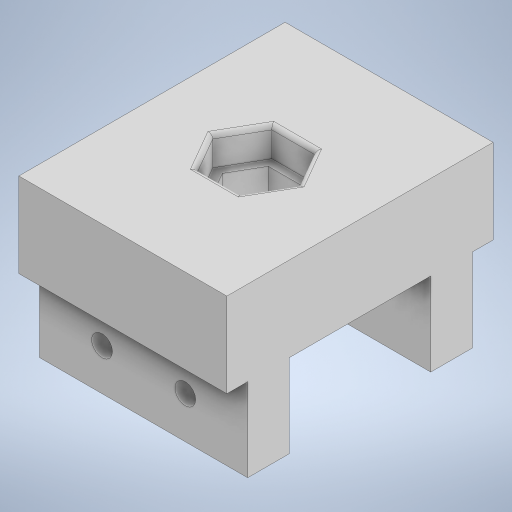
# Autodesk Inventor part: Tensile_test_bottom_adapter2
Saved by Autodesk Inventor 2024 (Build 280153000, 153)
## iProperties
Created: 2023-10-26
Part Number: Tensile_test_bottom_adapter2
Material: 일반
Document SubType Name: Modeling
Designer: jsw
Density: 1 g/cm^3
Appearance: 기본값
Author: jsw
Autodesk Inventor part; units mm, degrees
ref_plane "YZ Plane" through (0, 0, 0) normal (1, 0, 0) x (0, 1, 0)
ref_plane "XZ Plane" through (0, 0, 0) normal (0, 1, 0) x (-1, 0, 0)
ref_plane "XY Plane" through (0, 0, 0) normal (0, 0, 1) x (1, 0, 0)
sketch "스케치1" plane through (0, 0, 0) normal (0, 1, 0) x (-1, 0, 0)
  line L0 (-12.5, 16) -> (12.5, 16)
  line L1 (12.5, 16) -> (12.5, -16)
  line L2 (12.5, -16) -> (-12.5, -16)
  line L3 (-12.5, -16) -> (-12.5, 16)
  line L4 (-12.5, 16) -> (12.5, -16) construction
  line L5 (12.5, 16) -> (-12.5, -16) construction
  point P0 (0, 0)
  dimension "d0" = 25
  dimension "d1" = 32
  constraints: 12 end point, 2 midpoint, 2 parallel, 1 horizontal, 1 perpendicular
  measures "d0" distance of L1.end L2.end
  measures "d1" distance of L0.end L1.end
extrude "돌출1" add sketch "스케치1" along normal blind 10.16
sketch "스케치4" plane through (0, 0, 0) normal (0, -1, 0) x (1, 0, 0)
  line L0 (-12.5, -16) -> (-12.5, 16) projected
  line L1 (12.5, 16) -> (12.5, -16) projected
  line L2 (-12.5, 13.5) -> (12.5, 13.5)
  line L3 (12.5, 13.5) -> (12.5, 8.5)
  line L4 (12.5, 8.5) -> (-12.5, 8.5)
  line L5 (-12.5, 8.5) -> (-12.5, 13.5)
  line L6 (-12.5, 0) -> (12.5, 0)
  line L7 (-12.5, 16) -> (-12.5, -16)
  line L8 (12.5, -10.8) -> (12.5, 10.8)
  line L9 (-12.5, -13.5) -> (12.5, -13.5)
  line L10 (12.5, -13.5) -> (12.5, -8.5)
  line L11 (12.5, -8.5) -> (-12.5, -8.5)
  line L12 (-12.5, -8.5) -> (-12.5, -13.5)
  point P0 (0, 0)
  point P1 (12.5, -8.5)
  point P2 (-12.5, -13.5)
  point P3 (12.5, -13.5)
  point P4 (12.5, 13.5)
  dimension "d13" = 8.5
  dimension "d14" = 5
  constraints: 22 end point, 8 symmetric about line, 4 point on line, 2 midpoint, 2 parallel, 1 horizontal, 1 perpendicular
  measures "d13" distance from line of point (0, 0) L4
  measures "d14" distance of L2.end L3.end
extrude "돌출4" add sketch "스케치4" along normal blind 10 contours L0 L11 L1 L9 | L0 L2 L1 L4
sketch "스케치5" plane through (12.5, 0, -13.5) normal (0, 0, -1) x (-1, 0, 0)
  circle A0 centre (17.5, -5) radius 1.25
  line L0 (25, -10) -> (0, -10) projected
  line L1 (25, 0) -> (25, -10) projected
  line L2 (12.5, -10) -> (12.5, 0)
  circle A1 centre (7.5, -5) radius 1.25
  dimension "d17" = 2.5
  dimension "d18" = 5
  dimension "d22" = 5
  constraints: 2 centre point, 2 end point, 1 midpoint, 1 symmetric about line, 1 vertical, 1 other
  measures "d17" diameter of A0
  measures "d18" distance from line of A0.centre L0
  measures "d22" distance from line of L2 A0.centre
extrude "돌출5" cut sketch "스케치5" against normal up to surface (27 mm away)
sketch "스케치6" plane through (0, 10.16, 0) normal (0, 1, 0) x (1, 0, 0)
  circle A0 centre (0, 0) radius 4.5
  line L0 (2.5981, -4.5) -> (-2.5981, -4.5)
  line L1 (-2.5981, -4.5) -> (-5.1962, 0)
  line L2 (-5.1962, 0) -> (-2.5981, 4.5)
  line L3 (-2.5981, 4.5) -> (2.5981, 4.5)
  line L4 (2.5981, 4.5) -> (5.1962, 0)
  line L5 (5.1962, 0) -> (2.5981, -4.5)
  dimension "d25" = 9
  constraints: 12 end point, 2 coincident, 1 centre point, 1 horizontal, 1 tangent, 13 other
  measures "d25" diameter of A0
extrude "돌출6" cut sketch "스케치6" against normal blind 8
sketch "스케치7" plane through (0, 2.16, 0) normal (0, 1, 0) x (1, 0, 0)
  line L0 (2.5981, 4.5) -> (5.1962, 0) projected
  line L1 (-2.5981, 4.5) -> (2.5981, 4.5) projected
  line L2 (-5.1962, 0) -> (-2.5981, 4.5) projected
  line L3 (-2.5981, -4.5) -> (-5.1962, 0) projected
  line L4 (2.5981, -4.5) -> (-2.5981, -4.5) projected
  line L5 (5.1962, 0) -> (2.5981, -4.5) projected
  line L6 (-2.0207, 3.5) -> (2.0207, 3.5)
  line L7 (2.0207, 3.5) -> (4.0415, 0)
  line L8 (4.0415, 0) -> (2.0207, -3.5)
  line L9 (2.0207, -3.5) -> (-2.0207, -3.5)
  line L10 (-2.0207, -3.5) -> (-4.0415, 0)
  line L11 (-4.0415, 0) -> (-2.0207, 3.5)
  point P0 (0, 0)
  point P1 (0, 0)
  dimension "d29" = 1
  constraints: 12 end point, 1 coincident, 1 horizontal, 13 other
  measures "d29" distance between parallel lines of L11 L2
extrude "돌출7" add sketch "스케치7" along normal blind 4.5
fillet "모깎기1" radius 0.5 6 edges at (-3.8971, 10.16, 2.25) (0, 10.16, 4.5) (-3.8971, 10.16, -2.25) (0, 10.16, -4.5) (3.8971, 10.16, -2.25) (3.8971, 10.16, 2.25)
